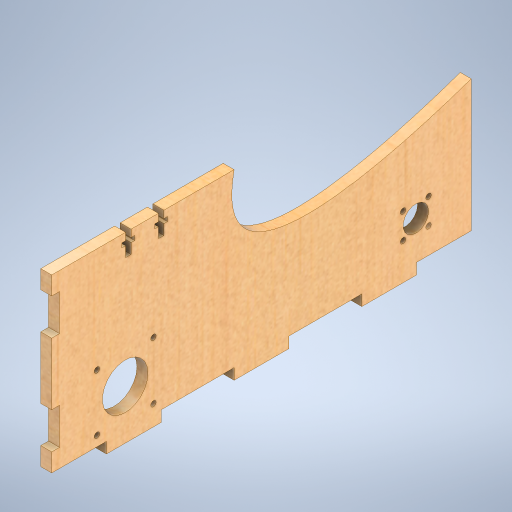
# Autodesk Inventor part: бок
Saved by Autodesk Inventor 2024.2 (Build 282272000, 272)
## iProperties
Created: 2026-01-28
Part Number: бок
Material: Типовые
Document SubType Name: Modeling
Designer: Zakhar
Density: 1 g/cm^3
Appearance: Желтая сосна — массив — светлое морение — со слабым глянцем
Author: Zakhar
Autodesk Inventor part; units mm, degrees
ref_plane "YZ Plane" through (0, 0, 0) normal (1, 0, 0) x (0, 1, 0)
ref_plane "XZ Plane" through (0, 0, 0) normal (0, 1, 0) x (-1, 0, 0)
ref_plane "XY Plane" through (0, 0, 0) normal (0, 0, 1) x (1, 0, 0)
sketch "Эскиз1" plane through (0, 0, 0) normal (1, 0, 0) x (0, 1, 0)
  line L0 (35.7991, 182.11) -> (-64.2009, 182.11)
  line L1 (-64.2009, 182.11) -> (-64.2009, -47.89)
  line L2 (-64.2009, -47.89) -> (35.7991, -47.89)
  line L3 (35.7991, -47.89) -> (35.7991, 182.11)
  spline S0 degree 3 poles (35.7991, 82.11) (-39.3426, 97.9096) (5.4101, -36.8502) (35.7991, -101.803) knots 0 0 0 0 1 1 1 1
  point P0 (0, 0)
  point P1 (-0.0002, 69.5066)
  point P2 (13.9408, -47.89)
  dimension "d0" = 230
  dimension "d1" = 100
  dimension "d20" = 100
  constraints: 8 end point, 2 parallel, 2 point on line, 1 horizontal, 1 perpendicular, 4 other
  measures "d0" distance of L0.end L1.end
  measures "d1" distance of L0.start L0.end
  measures "d20" distance from line of L0 point (35.799, 82.11)
extrude "Выдавливание1" add sketch "Эскиз1" along normal blind 6 contours L3 S0 L2 L1 L0
sketch "Эскиз2" plane through (6, 0, 0) normal (1, 0, 0) x (0, 0, -1)
  line L0 (-182.11, 35.7991) -> (-182.11, -64.2009) projected
  line L1 (-182.11, -64.2009) -> (47.89, -64.2009) projected
  line L2 (-182.11, -58.2009) -> (-152.11, -58.2009)
  line L3 (-152.11, -58.2009) -> (-152.11, -64.2009)
  line L4 (-152.11, -64.2009) -> (-182.11, -64.2009)
  line L5 (-182.11, -64.2009) -> (-182.11, -58.2009)
  line L6 (-152.11, -58.2009) -> (-122.11, -58.2009)
  line L7 (-122.11, -58.2009) -> (-122.11, -64.2009)
  line L8 (-122.11, -64.2009) -> (-152.11, -64.2009)
  line L9 (-152.11, -64.2009) -> (-152.11, -58.2009)
  line L10 (-122.11, -58.2009) -> (-82.11, -58.2009)
  line L11 (-82.11, -58.2009) -> (-82.11, -64.2009)
  line L12 (-82.11, -64.2009) -> (-122.11, -64.2009)
  line L13 (-122.11, -64.2009) -> (-122.11, -58.2009)
  line L14 (47.89, -64.2009) -> (47.89, 13.9408) projected
  line L15 (47.89, -58.2009) -> (17.89, -58.2009)
  line L16 (17.89, -58.2009) -> (17.89, -64.2009)
  line L17 (17.89, -64.2009) -> (47.89, -64.2009)
  line L18 (47.89, -64.2009) -> (47.89, -58.2009)
  line L19 (17.89, -58.2009) -> (-12.11, -58.2009)
  line L20 (-12.11, -58.2009) -> (-12.11, -64.2009)
  line L21 (-12.11, -64.2009) -> (17.89, -64.2009)
  line L22 (17.89, -64.2009) -> (17.89, -58.2009)
  line L23 (-12.11, -58.2009) -> (-52.11, -58.2009)
  line L24 (-52.11, -58.2009) -> (-52.11, -64.2009)
  line L25 (-52.11, -64.2009) -> (-12.11, -64.2009)
  line L26 (-12.11, -64.2009) -> (-12.11, -58.2009)
  line L27 (-52.11, -58.2009) -> (-82.11, -58.2009)
  line L28 (-82.11, -58.2009) -> (-82.11, -64.2009)
  line L29 (-82.11, -64.2009) -> (-52.11, -64.2009)
  line L30 (-52.11, -64.2009) -> (-52.11, -58.2009)
  point P0 (0, 0)
  point P1 (47.89, 35.7991)
  point P2 (-122.11, -64.2009)
  dimension "d4" = 30
  dimension "d5" = 30
  dimension "d6" = 40
  dimension "d7" = 30
  dimension "d8" = 30
  dimension "d9" = 40
  dimension "d12" = 6
  dimension "d13" = 6
  constraints: 56 end point, 14 parallel, 8 point on line, 7 horizontal, 7 perpendicular
  measures "d4" distance of L2.start L2.end
  measures "d5" distance of L2.end L6.end
  measures "d6" distance of L6.end L10.end
  measures "d7" distance of L15.start L15.end
  measures "d8" distance of L15.end L19.end
  measures "d9" distance of L19.end L23.end
  measures "d12" distance of L2.end L3.end
  measures "d13" distance of L27.end L11.end
extrude "Выдавливание2" cut sketch "Эскиз2" against normal through all contours L2 L3 L1 L0 | L10 L11 L1 L7 | L23 L20 L1 L24 | L15 L14 L1 L16
sketch "Эскиз3" plane through (0, 0, 0) normal (-1, 0, 0) x (0, 0, 1)
  line L0 (182.11, -58.2009) -> (177.838, -58.2009)
  line L1 (177.838, -58.2009) -> (177.838, -48.2009)
  line L2 (177.838, -48.2009) -> (182.11, -48.2009)
  line L3 (182.11, -48.2009) -> (182.11, -58.2009)
  line L4 (177.838, -48.2009) -> (182.11, -48.2009)
  line L5 (182.11, -48.2009) -> (182.11, -28.2009)
  line L6 (182.11, -28.2009) -> (177.838, -28.2009)
  line L7 (177.838, -28.2009) -> (177.838, -48.2009)
  line L8 (182.11, -28.2009) -> (177.838, -28.2009)
  line L9 (177.838, -28.2009) -> (177.838, 5.7991)
  line L10 (177.838, 5.7991) -> (182.11, 5.7991)
  line L11 (182.11, 5.7991) -> (182.11, -28.2009)
  line L12 (177.838, 5.7991) -> (182.11, 5.7991)
  line L13 (182.11, 5.7991) -> (182.11, 25.7991)
  line L14 (182.11, 25.7991) -> (177.838, 25.7991)
  line L15 (177.838, 25.7991) -> (177.838, 5.7991)
  line L16 (182.11, 35.7991) -> (182.11, -58.2009) projected
  line L17 (177.838, 25.7991) -> (182.11, 25.7991)
  line L18 (182.11, 25.7991) -> (182.11, 35.7991)
  line L19 (182.11, 35.7991) -> (177.838, 35.7991)
  line L20 (177.838, 35.7991) -> (177.838, 25.7991)
  point P0 (0, 0)
  dimension "d14" = 10
  dimension "d15" = 10
  dimension "d16" = 20
  dimension "d17" = 20
  constraints: 40 end point, 10 parallel, 5 horizontal, 5 perpendicular, 3 point on line
  measures "d14" distance of L0.end L1.end
  measures "d15" distance of L19.end L14.end
  measures "d16" distance of L6.end L1.end
  measures "d17" distance of L14.end L9.end
extrude "Выдавливание3" cut sketch "Эскиз3" against normal blind 6 contours L2 L7 L6 L5 | L10 L15 L14 L13
sketch "Эскиз4" plane through (6, 0, 0) normal (1, 0, 0) x (0, 0, -1)
  line L0 (-162.838, -58.2009) -> (-120.838, -58.2009)
  line L1 (-120.838, -58.2009) -> (-120.838, -50.2009)
  line L2 (-120.838, -50.2009) -> (-162.838, -50.2009)
  line L3 (-162.838, -50.2009) -> (-162.838, -58.2009)
  line L4 (-120.838, -58.2009) -> (-128.838, -58.2009)
  line L5 (-128.838, -58.2009) -> (-128.838, -16.2009)
  line L6 (-128.838, -16.2009) -> (-120.838, -16.2009)
  line L7 (-120.838, -16.2009) -> (-120.838, -58.2009)
  line L8 (-120.838, -16.2009) -> (-162.838, -16.2009)
  line L9 (-162.838, -16.2009) -> (-162.838, -24.2009)
  line L10 (-162.838, -24.2009) -> (-120.838, -24.2009)
  line L11 (-120.838, -24.2009) -> (-120.838, -16.2009)
  line L12 (-162.838, -16.2009) -> (-154.838, -16.2009)
  line L13 (-154.838, -16.2009) -> (-154.838, -58.2009)
  line L14 (-154.838, -58.2009) -> (-162.838, -58.2009)
  line L15 (-162.838, -58.2009) -> (-162.838, -16.2009)
  line L16 (-162.838, -45.8935) -> (-162.838, -53.8935)
  circle A0 centre (-157.338, -21.7009) radius 1.5
  circle A1 centre (-126.338, -21.7009) radius 1.5
  circle A2 centre (-126.338, -53.2009) radius 1.5
  circle A3 centre (-157.338, -52.7009) radius 1.5
  circle A4 centre (-141.838, -37.2009) radius 12.5
  line L17 (-182.11, -58.2009) -> (-152.11, -58.2009) projected
  line L18 (-177.838, -28.2009) -> (-177.838, -48.2009) projected
  circle A5 centre (17.497, -37.2009) radius 7
  circle A6 centre (10.497, -30.2009) radius 1.5
  circle A7 centre (24.497, -30.2009) radius 1.5
  circle A8 centre (24.497, -44.2009) radius 1.5
  circle A9 centre (10.497, -44.2009) radius 1.5
  line L19 (24.497, -30.2009) -> (24.497, -44.2009) construction
  line L20 (24.497, -44.2009) -> (10.497, -44.2009) construction
  line L21 (10.497, -30.2009) -> (10.497, -44.2009) construction
  line L22 (10.497, -30.2009) -> (24.497, -30.2009) construction
  point P0 (0, 0)
  point P1 (-141.838, -58.2009)
  point P2 (-176.8137, 14.1065)
  point P3 (-162.838, -53.8935)
  point P4 (-162.838, -45.8935)
  point P5 (4.035, -43.7767)
  point P6 (21.9204, -26.629)
  dimension "d21" = 42
  dimension "d22" = 42
  dimension "d23" = 8
  dimension "d24" = 8
  dimension "d25" = 8
  dimension "d26" = 8
  dimension "d27" = 3
  dimension "d28" = 3
  dimension "d29" = 3
  dimension "d30" = 3
  dimension "d31" = 5.5
  dimension "d32" = 5.5
  dimension "d33" = 5.5
  dimension "d34" = 5.5
  dimension "d35" = 5.5
  dimension "d36" = 5.5
  dimension "d37" = 5.5
  dimension "d38" = 21
  dimension "d39" = 21
  dimension "d40" = 25
  dimension "d41" = 3
  dimension "d42" = 15
  dimension "d45" = 14
  dimension "d46" = 3
  dimension "d47" = 3
  dimension "d48" = 3
  dimension "d49" = 3
  constraints: 40 end point, 10 centre point, 8 parallel, 7 perpendicular, 4 horizontal, 4 tangent, 2 point on line, 2 vertical, 1 collinear, 1 midpoint, 3 other
  measures "d21" distance of L10.start L11.start
  measures "d22" distance of L14.end L8.end
  measures "d23" distance between parallel lines of L8 L10
  measures "d24" distance between parallel lines of L7 L5
  measures "d25" distance from line of point (-141.838, -58.201) L2
  measures "d26" distance between parallel lines of L15 L13
  measures "d27" diameter of A0
  measures "d28" diameter of A1
  measures "d29" diameter of A2
  measures "d30" diameter of A3
  measures "d31" distance from line of L0 A3.centre
  measures "d32" distance from line of L15 A3.centre
  measures "d33" distance from line of L7 A2.centre
  measures "d34" distance from line of L11 A1.centre
  measures "d35" distance from line of L6 A1.centre
  measures "d36" distance from line of L8 A0.centre
  measures "d37" distance from line of L9 A0.centre
  measures "d38" distance of point (-141.838, -58.201) A4.centre
  measures "d39" distance from line of L15 A4.centre
  measures "d40" diameter of A4
  measures "d41" distance from line of L2 A2.centre
  measures "d42" distance between parallel lines of L18 L15
  measures "d45" diameter of A5
  measures "d46" diameter of A6
  measures "d47" diameter of A7
  measures "d48" diameter of A8
  measures "d49" diameter of A9
extrude "Выдавливание4" cut sketch "Эскиз4" against normal blind 6 contours A0 | A1 | A2 | A3 | A4 | A5 | A6 | A7 | A8 | A9
sketch "Эскиз5" plane through (6, 0, 0) normal (1, 0, 0) x (0, 0, -1)
  line L0 (-82.11, 35.7991) -> (-182.11, 35.7991) projected
  line L1 (-141.61, 35.7991) -> (-138.61, 35.7991)
  line L2 (-138.61, 35.7991) -> (-138.61, 23.7991)
  line L3 (-138.61, 23.7991) -> (-141.61, 23.7991)
  line L4 (-141.61, 23.7991) -> (-141.61, 35.7991)
  line L5 (-136.61, 29.3991) -> (-143.61, 29.3991)
  line L6 (-143.61, 29.3991) -> (-143.61, 31.7991)
  line L7 (-143.61, 31.7991) -> (-136.61, 31.7991)
  line L8 (-136.61, 31.7991) -> (-136.61, 29.3991)
  line L9 (-182.11, 35.7991) -> (-182.11, 25.7991) projected
  line L10 (-123.61, 35.7991) -> (-120.61, 35.7991)
  line L11 (-120.61, 35.7991) -> (-120.61, 23.7991)
  line L12 (-120.61, 23.7991) -> (-123.61, 23.7991)
  line L13 (-123.61, 23.7991) -> (-123.61, 35.7991)
  line L14 (-118.61, 29.3991) -> (-125.61, 29.3991)
  line L15 (-125.61, 29.3991) -> (-125.61, 31.7991)
  line L16 (-125.61, 31.7991) -> (-118.61, 31.7991)
  line L17 (-118.61, 31.7991) -> (-118.61, 29.3991)
  line L18 (-82.11, 35.7991) -> (-182.11, 35.7991) projected
  point P0 (0, 0)
  point P1 (-143.61, 30.5991)
  point P2 (-125.61, 30.5991)
  point P3 (-120.61, 29.3991)
  point P4 (-120.61, 31.7991)
  point P5 (-123.61, 31.7991)
  point P6 (-123.61, 29.3991)
  point P7 (-138.61, 31.7991)
  point P8 (-138.61, 35.7991)
  point P9 (-141.61, 31.7991)
  point P10 (-141.61, 29.3991)
  point P11 (-138.61, 29.3991)
  dimension "d50" = 3
  dimension "d51" = 2.4
  dimension "d52" = 7
  dimension "d53" = 2
  dimension "d54" = 12
  dimension "d55" = 4
  dimension "d56" = 38.5
  dimension "d57" = 3
  dimension "d58" = 2.4
  dimension "d59" = 7
  dimension "d60" = 2
  dimension "d61" = 12
  dimension "d63" = 38.5
  constraints: 32 end point, 8 parallel, 4 horizontal, 4 perpendicular, 2 collinear, 2 midpoint, 1 point on line
  measures "d50" distance of L2.end L3.end
  measures "d51" distance between parallel lines of L7 L5
  measures "d52" distance of L6.end L7.end
  measures "d53" distance between parallel lines of L4 L6
  measures "d54" distance of L1.end L2.end
  measures "d55" distance between parallel lines of L0 L7
  measures "d56" distance from line of L9 point (-143.61, 30.599)
  measures "d57" distance of L11.end L12.end
  measures "d58" distance between parallel lines of L16 L14
  measures "d59" distance of L15.end L16.end
  measures "d60" distance between parallel lines of L13 L15
  measures "d61" distance of L10.end L11.end
  measures "d63" distance from line of L11 L0.start
extrude "Выдавливание5" cut sketch "Эскиз5" against normal through all
equation "\"d28\" = d27"
equation "\"d29\" = d27"
equation "\"d30\" = d27"
